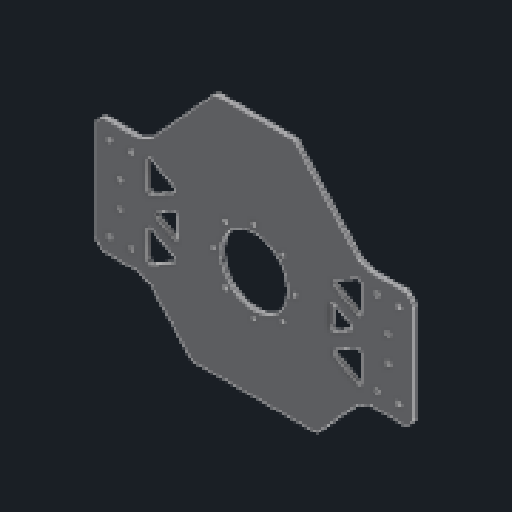
# Autodesk Inventor part: Root
Saved by Autodesk Inventor 2025.2 (Build 292293000, 293)
## iProperties
Created: 2020-05-07
Part Number: Root
Material: Generic
Document SubType Name: Sheet Metal
Designer: valer
Density: 1 g/cm^3
Sheet Metal Rule: Default
Appearance: Default
Author: valer
Autodesk Inventor part; units mm, degrees
ref_plane "YZ Plane" through (0, 0, 0) normal (1, 0, 0) x (0, 1, 0)
ref_plane "XZ Plane" through (0, 0, 0) normal (0, 1, 0) x (-1, 0, 0)
ref_plane "XY Plane" through (0, 0, 0) normal (0, 0, 1) x (1, 0, 0)
sketch "Base" plane through (0, 0, 0) normal (0, 0, 1) x (1, 0, 0)
  circle A0 centre (-56.25, 0) radius 2.75 construction
  circle A1 centre (0, -56.25) radius 2.75 construction
  circle A2 centre (0, 56.25) radius 2.75 construction
  circle A3 centre (39.7748, -39.7748) radius 2.75 construction
  circle A4 centre (-39.7748, 39.7748) radius 2.75 construction
  circle A5 centre (-39.7748, -39.7748) radius 2.75 construction
  circle A6 centre (39.7748, 39.7748) radius 2.75 construction
  circle A7 centre (56.25, 0) radius 2.75 construction
  circle A8 centre (0, 0) radius 45 construction
  circle A9 centre (0, 0) radius 61
  line L0 (220, 80) -> (-220, 80) construction
  line L1 (0, -210) -> (0, 210) construction
  line L2 (-308, 0) -> (308, 0) construction
  line L3 (-220, 80) -> (-150, 80)
  line L4 (-150, 80) -> (-150, 0)
  line L5 (-150, 0) -> (-220, 0)
  line L6 (-220, 0) -> (-220, 80)
  line L7 (86.6025, -150) -> (-86.6025, -150)
  line L8 (-86.6025, -150) -> (-173.2051, 0)
  line L9 (-173.2051, 0) -> (-86.6025, 150)
  line L10 (-86.6025, 150) -> (86.6025, 150)
  line L11 (86.6025, 150) -> (173.2051, 0)
  line L12 (173.2051, 0) -> (86.6025, -150)
  line L13 (-150, 0) -> (-86.6025, 150) construction
  line L14 (220, 80) -> (150, 80)
  line L15 (150, 80) -> (150, 0)
  line L16 (150, 0) -> (220, 0)
  line L17 (220, 0) -> (220, 80)
  line L18 (150, 0) -> (86.6025, 150) construction
  line L19 (-220, -80) -> (-150, -80)
  line L20 (-150, -80) -> (-150, 0)
  line L21 (-150, 0) -> (-219.7895, 0)
  line L22 (-219.7895, 0) -> (-220, -80)
  line L23 (-150, 0) -> (-86.6025, -150) construction
  line L24 (220, 0) -> (220, -80)
  line L25 (220, -80) -> (150, -80)
  line L26 (150, -80) -> (150, 0)
  line L27 (150, 0) -> (220, 0)
  line L28 (150, 0) -> (86.6025, -150) construction
  circle A10 centre (0, 0) radius 46.5
  circle A11 centre (-56.25, 0) radius 2.25
  circle A12 centre (-39.7748, -39.7748) radius 2.25
  circle A13 centre (0, -56.25) radius 2.25
  circle A14 centre (39.7748, -39.7748) radius 2.25
  circle A15 centre (56.25, 0) radius 2.25
  circle A16 centre (39.7748, 39.7748) radius 2.25
  circle A17 centre (0, 56.25) radius 2.25
  circle A18 centre (-39.7748, 39.7748) radius 2.25
  line L29 (-150, 80) -> (-86.6025, 150)
  line L30 (86.6025, 150) -> (150, 80)
  line L31 (-150, -80) -> (-86.6025, -150)
  line L32 (86.6025, -150) -> (150, -80)
  point P0 (0, 0)
  point P1 (210, 0)
  point P2 (150, 40.1924)
  point P3 (150, -40.1924)
  point P4 (173.2051, 0)
  point P5 (173.2051, 0)
  point P6 (-150, 40.1924)
  point P7 (-173.2051, 0)
  point P8 (-173.2051, 0)
  point P9 (-150, -40.1924)
  point P10 (173.2051, 0)
  point P11 (-173.2051, 0)
  point P12 (-173.2051, 0)
  dimension "d89" = 80
  dimension "d90" = 70
  dimension "d91" = 1.5
  dimension "d92" = 4.5
  dimension "d157" = 150
  dimension "d158" = 220
  measures "d89" distance between parallel lines of L0 L5
  measures "d90" distance between parallel lines of L4 L6
  measures "d91" radial gap between concentric circles of A10 A8
  measures "d92" diameter of A11
  measures "d157" distance from line of L7 A8.centre
  measures "d158" distance between parallel lines of L24 L1
extrude "Plate1" add sketch "Base" against normal blind 5 contours A9 | L3 L4 L9 L5 L6 | L29 L9 L4 | L9 L10 L11 L15 L26 L12 L7 L8 L20 L4 | L4 L5 L9 | L5 L8 L20 L19 L22 | L20 L8 L5 | L30 L15 L11 | L8 L31 L20 | L15 L14 L17 L16 L11 | L11 L16 L15 | L16 L24 L25 L26 L12 | L12 L26 L16 | L12 L26 L32
sketch "LegMountHoles" plane through (0, 0, -5) normal (0, 0, -1) x (-1, 0, 0)
  line L0 (-222.4542, 0) -> (-220, 0) construction
  line L1 (-220, 80) -> (-150, 80) construction
  line L2 (-185, 80) -> (-185, 0) construction
  line L3 (-170, 58) -> (-200, 58) construction
  circle A0 centre (-170, 58) radius 3
  circle A1 centre (-200, 58) radius 3
  circle A2 centre (-185, 18) radius 3
  line L4 (308.4908, 0) -> (-310.9451, 0) construction
  line L5 (0, -210) -> (0, 210) construction
  circle A3 centre (170, 58) radius 3
  circle A4 centre (200, 58) radius 3
  circle A5 centre (185, 18) radius 3
  circle A6 centre (-170, -58) radius 3
  circle A7 centre (-200, -58) radius 3
  circle A8 centre (-185, -18) radius 3
  circle A9 centre (170, -58) radius 3
  circle A10 centre (200, -58) radius 3
  circle A11 centre (185, -18) radius 3
  line L6 (-150, 80) -> (-86.6025, 150) projected
  line L7 (-220, -80) -> (-220, 80) projected
  point P0 (0, 0)
  point P1 (-185, 58)
  dimension "d93" = 6
  dimension "d94" = 30
  dimension "d95" = 40
  dimension "d161" = 18
  constraints: 12 centre point, 9 symmetric about line, 6 end point, 4 point on line, 2 coincident, 2 equal radius, 2 horizontal, 2 midpoint, 2 perpendicular, 1 collinear, 9 other
  measures "d93" diameter of A0
  measures "d94" distance of L3.start L3.end
  measures "d95" distance from line of L3 A2.centre
  measures "d161" distance from line of L4 A2.centre
extrude "LegMountHolesFeature" cut sketch "LegMountHoles" against normal blind 5
chamfer "OutsideChamfersFeature" distance 10 angle 45 8 edges at (-220, -80, -2.5) (-150, -80, -2.5) (150, -80, -2.5) (220, -80, -2.5) (-220, 80, -2.5) (-150, 80, -2.5) (150, 80, -2.5) (220, 80, -2.5)
fillet "OutsideFilletsFeature" radius 8 18 edges at (160, 80, -2.5) (210, 80, -2.5) (220, 70, -2.5) (210, -80, -2.5) (160, -80, -2.5) (86.6025, -150, -2.5) (-86.6025, -150, -2.5) (-160, -80, -2.5) (-210, -80, -2.5) (-219.9737, -70, -2.5) (-220, 0, -2.5) (-220, 70, -2.5) (-210, 80, -2.5) (-160, 80, -2.5) (-143.2871, 87.412, -2.5) (143.2871, 87.412, -2.5) (143.2871, -87.412, -2.5) (-143.2871, -87.412, -2.5)
sketch "LaserMount" plane through (0, 0, -5) normal (0, 0, -1) x (-1, 0, 0)
  line L0 (86.6025, 150) -> (142.1497, 88.6679)
  line L1 (86.6025, 150) -> (54.9038, 185)
  line L2 (54.9038, 185) -> (0, 185)
  line L3 (0, -217) -> (0, 252) construction
  line L4 (-86.6025, 150) -> (86.6025, 150)
  line L5 (-86.6025, 150) -> (-54.9038, 185)
  line L6 (-54.9038, 185) -> (0, 185)
  line L7 (86.6025, 150) -> (142.1497, 88.6679)
  point P0 (0, 0)
  dimension "d119" = 35
  measures "d119" distance between parallel lines of L2 L4
sheet face with bend "LaserMountFeature" sketch "LaserMount" thickness 5 toward (0, 0, 1) bend radius 5 relief straight relief width 5 relief depth 2.5
bend "Bend4"
fillet "FrontFilletsFeature" radius 8 2 edges at (-54.9038, 185, -2.5) (54.9038, 185, -2.5)
sketch "TrianglePattern" plane through (0, 0, -5) normal (0, 0, -1) x (-1, 0, 0)
  line L0 (-148.3013, -66.7074) -> (-105, -41.7074)
  line L1 (-105, -41.7074) -> (-148.3013, -16.7074)
  line L2 (-148.3013, -16.7074) -> (-148.3013, -66.7074)
  line L3 (-139.641, 0) -> (-105, -20)
  line L4 (-105, -20) -> (-105, 20)
  line L5 (-105, 20) -> (-139.641, 0)
  line L6 (308, 0) -> (-308, 0) construction
  line L7 (-148.3013, 66.7074) -> (-105, 41.7074)
  line L8 (-105, 41.7074) -> (-148.3013, 16.7074)
  line L9 (-148.3013, 16.7074) -> (-148.3013, 66.7074)
  line L10 (0, -217) -> (0, 252) construction
  line L11 (148.3013, -66.7074) -> (105, -41.7074)
  line L12 (105, -41.7074) -> (148.3013, -16.7074)
  line L13 (148.3013, -16.7074) -> (148.3013, -66.7074)
  line L14 (139.641, 0) -> (105, -20)
  line L15 (105, -20) -> (105, 20)
  line L16 (105, 20) -> (139.641, 0)
  line L17 (148.3013, 16.7074) -> (148.3013, 66.7074)
  line L18 (148.3013, 66.7074) -> (105, 41.7074)
  line L19 (105, 41.7074) -> (148.3013, 16.7074)
  line L20 (-105, 41.7074) -> (-105, 20) construction
  line L21 (-105, 41.7074) -> (-148.3013, 41.7074) construction
  line L22 (-105, -41.7074) -> (-148.3013, -41.7074) construction
  point P0 (0, 0)
  dimension "d149" = 30
  dimension "d150" = 18.7992
  dimension "d151" = 30
  dimension "d152" = 30
  dimension "d153" = 18.7992
  dimension "d154" = 40
  dimension "d155" = 50
  dimension "d156" = 105
  constraints: 42 end point, 12 symmetric about line, 4 parallel, 2 midpoint, 1 collinear, 1 perpendicular, 1 point on line
  measures "d149" angle of L6 L5
  measures "d150" distance between parallel lines of L5 L8
  measures "d151" angle of L8 L21
  measures "d152" angle of L22 L1
  measures "d153" distance between parallel lines of L1 L3
  measures "d154" distance of L3.end L4.end
  measures "d155" distance of L9.start L9.end
  measures "d156" distance from line of L4 point (0, 0)
extrude "TriangleHolesFeature" cut sketch "TrianglePattern" against normal blind 5
fillet "TriangleHoleFilletsFeature" radius 4 18 edges at (105, -20, -2.5) (105, 20, -2.5) (139.641, 0, -2.5) (105, -41.7074, -2.5) (148.3013, -16.7074, -2.5) (148.3013, -66.7074, -2.5) (105, 41.7074, -2.5) (148.3013, 66.7074, -2.5) (148.3013, 16.7074, -2.5) (-148.3013, 66.7074, -2.5) (-148.3013, 16.7074, -2.5) (-105, 41.7074, -2.5) (-139.641, 0, -2.5) (-105, 20, -2.5) (-105, -20, -2.5) (-148.3013, -16.7074, -2.5) (-148.3013, -66.7074, -2.5) (-105, -41.7074, -2.5)
equation "\"d97\" = Thickness"
equation "\"d33\" = Thickness"
equation "\"BendRadius\" = Thickness"
equation "\"BendReliefWidth\" = Thickness"
equation "\"BendReliefDepth\" = 0.5 * Thickness"
equation "\"TransitionRadius\" = BendRadius"
equation "\"JacobiRadiusSize\" = BendRadius"
equation "\"GapSize\" = Thickness"
equation "\"Thickness\" = 5"
body "Solid1"
